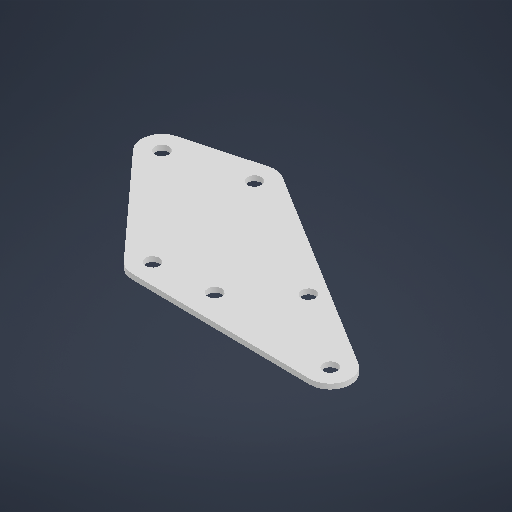
# Autodesk Inventor part: newsidepolytest
Saved by Autodesk Inventor 2025.2 (Build 292293000, 293)
## iProperties
Created: 2025-04-03
Part Number: newsidepolytest
Material: Generic
Document SubType Name: Modeling
Designer: Jahan
Density: 1 g/cm^3
Appearance: Default
Author: Jahan
Autodesk Inventor part; units mm, degrees
ref_plane "YZ Plane" through (0, 0, 0) normal (1, 0, 0) x (0, 1, 0)
ref_plane "XZ Plane" through (0, 0, 0) normal (0, 1, 0) x (-1, 0, 0)
ref_plane "XY Plane" through (0, 0, 0) normal (0, 0, 1) x (1, 0, 0)
sketch "Sketch1" plane through (0, 0, 0) normal (0, 1, 0) x (-1, 0, 0)
  circle A0 centre (-15.2763, 11.7192) radius 2.1844
  circle A1 centre (46.1983, -4.1823) radius 2.1844
  circle A2 centre (-0.2854, 25.8488) radius 2.1844
  circle A3 centre (17.6488, 27.2646) radius 2.1844
  circle A4 centre (23.5893, -10.3689) radius 2.1844
  circle A5 centre (-38.3261, 27.9733) radius 2.1844
  circle A6 centre (-38.3261, 27.9733) radius 6.35
  circle A7 centre (23.5893, -10.3689) radius 6.35
  line L0 (-41.6694, 22.5746) -> (20.246, -15.7676)
  circle A8 centre (17.6488, 27.2646) radius 6.35
  line L1 (17.7292, 33.6141) -> (-38.2458, 34.3228)
  circle A9 centre (46.1983, -4.1823) radius 6.35
  line L2 (50.8998, 0.086) -> (22.3503, 31.5329)
  line L3 (47.8742, -10.3072) -> (25.2652, -16.4937)
  point P0 (0, 0)
  point P1 (21.7554, 32.108)
  point P2 (24.1332, -16.6956)
  dimension "d0" = 12.7
  dimension "d1" = 12.7
  dimension "d2" = 12.7
  dimension "d10" = 12.7
  constraints: 10 centre point, 10 point on circle, 8 end point, 8 tangent, 4 coincident
  measures "d0" diameter of A6
  measures "d1" diameter of A7
  measures "d2" diameter of A8
  measures "d10" diameter of A9
extrude "Extrusion1" add sketch "Sketch1" along normal blind 1.5875
body "Solid1"
